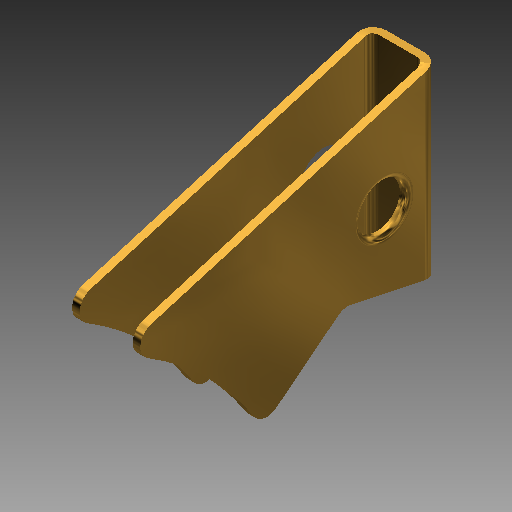
# Autodesk Inventor part: 403-03
Saved by Autodesk Inventor 2019 (Build 230136000, 136)
## iProperties
Company: Autodesk Inc.
Created: 2017-06-27
Part Number: 403-03
Material: Brass, Soft Yellow
Document SubType Name: Sheet Metal
Designer: Autodesk Inc.
Mass: 0.187874 g
Surface Area: 1.91783 cm^2
Volume: 0.0221811 cm^3
Density: 8.47 g/cm^3
Flat Pattern Width: 2.01491 cm
Flat Pattern Length: 0.904036 cm
Flat Pattern Area: 1.82156 cm^2
Sheet Metal Rule: Default_mm
Sheet Metal Width: 20.149 mm
Sheet Metal Length: 9.040 mm
Sheet Metal Area: 182.156 mm^2
Appearance: Brass - Satin
Author: Inventor
Autodesk Inventor part; units mm, degrees
ref_plane "YZ Plane" through (0, 0, 0) normal (1, 0, 0) x (0, 1, 0)
ref_plane "XZ Plane" through (0, 0, 0) normal (0, 1, 0) x (-1, 0, 0)
ref_plane "XY Plane" through (0, 0, 0) normal (0, 0, 1) x (1, 0, 0)
sketch "Sketch1" plane through (0, 0, 0) normal (0, 0, 1) x (1, 0, 0)
  line L0 (0, 0) -> (0, 6)
  line L1 (0, 6) -> (0.95, 6)
  line L2 (0.95, 6) -> (10.1278, 3.2814)
  arc A0 (10.2473, 2.3758) -> (10.1278, 3.2814) centre (9.9858, 2.802) ccw
  arc A1 (10.2473, 2.3758) -> (6.7696, -1.0168) centre (16, -7) ccw
  arc A2 (6.0402, -1.1372) -> (6.7696, -1.0168) centre (6.35, -0.7448) ccw
  line L3 (6.0402, -1.1372) -> (4.0098, 0.4658)
  arc A3 (4.0098, 0.4658) -> (3.596, 0.5624) centre (3.7, 0.0734) ccw
  line L4 (3.596, 0.5624) -> (0.95, 0)
  line L5 (0.95, 0) -> (0, 0)
  dimension "d0" = 6
  dimension "d1" = 0.95
  dimension "d2" = 3.7
  dimension "d3" = 11
  dimension "d4" = 16.5
  dimension "d5" = 0.5
  dimension "d6" = 16
  dimension "d7" = 13
  dimension "d8" = 12
  dimension "d33" = 6.35
  measures "d0" distance of L0.start L0.end
  measures "d1" distance of L0.end L1.end
  measures "d2" distance from line of A3.centre L0
  measures "d3" radius of A1
  measures "d4" angle of L1 L2
  measures "d5" radius of A3
  measures "d6" distance from line of L0 A1.centre
  measures "d7" distance from line of L1 A1.centre
  measures "d8" angle of L4 L5
  measures "d33" horizontal distance of A2.centre L0.start
extrude "Plate1" add sketch "Sketch1" against normal blind 0.25
sketch "Sketch2" plane through (0, 0, 0) normal (0, 0, 1) x (1, 0, 0)
  line L0 (0, 6) -> (0.95, 6) projected
  point P0 (0, 0)
  point P1 (2.5, 2.72)
  dimension "d10" = 3.28
  dimension "d11" = 2.5
  measures "d10" distance from line of point (2.5, 2.72) L0
  measures "d11" horizontal distance of L0.start point (2.5, 2.72)
hole "Hole1" at (2.5, 2.72, 0) direction (0, 0, -1) diameter 1.5 end through all
mirror "Mirror1" about plane through (0, 6, 0) normal (-1, 0, 0)
sketch "Sketch3" plane through (0, 0, 0) normal (0, 0, 1) x (1, 0, 0)
  line L0 (-0.9, 0) -> (-0.9, 6)
  line L1 (0.9, 6) -> (0.9, 0)
  line L2 (-0.9, 0) -> (0.9, 0) construction
  line L3 (0.95, 0) -> (-0.95, 0) projected
  line L4 (0.95, 6) -> (-0.95, 6) construction
  point P0 (0, 0)
  point P1 (0, 0)
  dimension "d19" = 1.8
  constraints: 6 end point, 2 midpoint, 2 point on line, 1 parallel, 1 perpendicular, 1 vertical
  measures "d19" distance of L0.start L1.end
fold "Fold1" angle 90 bend radius 0.25 thickness 0.25 k factor 0.44 line from (-0.9, 0, 0) to (-0.9, 6, 0) line at bend centre moving side (-1, 0, 0) folds toward (0, 0, 1)
fold "Fold2" angle 90 bend radius 0.25 thickness 0.25 k factor 0.44 line from (0.9, 6, 0) to (0.9, 0, 0) line at bend centre moving side (1, 0, 0) folds toward (0, 0, 1)
fillet "Fillet1" radius 0.2 2 edges at (-1.1173, 3.47, 1.5673) (1.1173, 3.47, 1.5673)
equation "\"d17\" = Thickness"
equation "\"d20\" = BendReliefWidth"
equation "\"d21\" = BendReliefDepth"
equation "\"d22\" = MinimumRemnant"
equation "\"d23\" = BendRadius"
equation "\"d32\" = Thickness"
equation "\"d26\" = BendReliefWidth"
equation "\"d27\" = BendReliefDepth"
equation "\"d28\" = MinimumRemnant"
equation "\"d29\" = BendRadius"
equation "\"BendRadius\" = Thickness"
equation "\"BendReliefDepth\" = 0.5 * Thickness"
equation "\"CornerReliefSize\" = 4 * Thickness"
equation "\"MinimumRemnant\" = 2 * Thickness"
equation "\"TransitionRadius\" = BendRadius"
equation "\"JacobiRadiusSize\" = BendRadius"
equation "\"GapSize\" = Thickness"
equation "\"d9\" = BendRadius"
equation "\"Thickness\" = 0.25"
equation "\"BendReliefWidth\" = 0.25"
body "Solid1"
